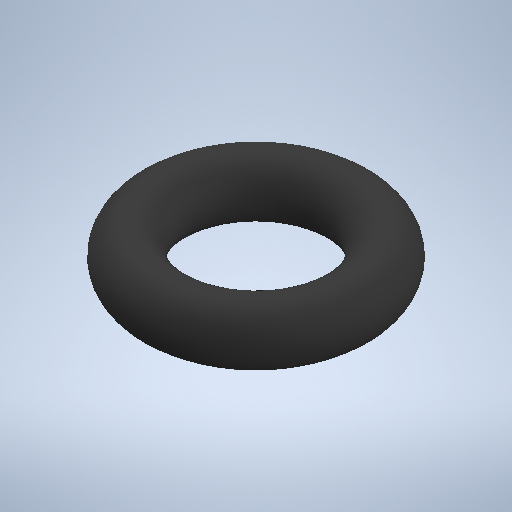
# Autodesk Inventor part: 12C VALVE BONNET SEAL
Saved by Autodesk Inventor 2025.2 (Build 292293000, 293)
## iProperties
Created: 2025-05-29
Part Number: 12C VALVE BONNET SEAL
Material: Rubber
Document SubType Name: Modeling
Designer: bless
Density: 0.93 g/cm^3
Appearance: Rubber - Black
Author: bless
Autodesk Inventor part; units mm, degrees
ref_plane "YZ Plane" through (0, 0, 0) normal (1, 0, 0) x (0, 1, 0)
ref_plane "XZ Plane" through (0, 0, 0) normal (0, 1, 0) x (-1, 0, 0)
ref_plane "XY Plane" through (0, 0, 0) normal (0, 0, 1) x (1, 0, 0)
sketch "Sketch1" plane through (0, 0, 0) normal (0, 0, 1) x (1, 0, 0)
  circle A0 centre (0, 0) radius 1.35
  line L0 (4.35, 2.1646) -> (4.35, -1.915) construction
  dimension "d0" = 1.35
  dimension "d1" = 5.7
  dimension "d2" = 4.8588
  dimension "d3" = 4.7529
  constraints: 2 end point, 1 centre point, 1 coincident, 1 vertical
  measures "d0" radius of A0
  measures "d2" distance of L0.start point (0, 0)
  measures "d3" distance of L0.end point (0, 0)
revolve "Revolution1" add sketch "Sketch1" angle 360 about axis through (4.35, 2.1646, 0) along (0, -1, 0)
body "Solid1"
